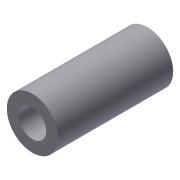
# Autodesk Inventor part: Toughbox Spacers
Saved by Autodesk Inventor 2011 (Build 150239000, 239)
## iProperties
Created: 2012-06-04
Part Number: Toughbox Spacers
Material: Aluminum-6061
Document SubType Name: Modeling
Designer: Nemo
Mass: 7.15711 g
Surface Area: 19.1779 cm^2
Volume: 2.641 cm^3
Density: 2.71 g/cm^3
Author: Nemo
Autodesk Inventor part; units mm, degrees
ref_plane "YZ Plane" through (0, 0, 0) normal (1, 0, 0) x (0, 1, 0)
ref_plane "XZ Plane" through (0, 0, 0) normal (0, 1, 0) x (-1, 0, 0)
ref_plane "XY Plane" through (0, 0, 0) normal (0, 0, 1) x (1, 0, 0)
sketch "Sketch1" plane through (0, 0, 0) normal (0, 0, 1) x (1, 0, 0)
  circle A0 centre (0, 0) radius 3.429
  circle A1 centre (0, 0) radius 6.35
  dimension "d0" = 6.858
  dimension "d1" = 12.7
  constraints: 2 centre point, 2 coincident
  measures "d0" diameter of A0
  measures "d1" diameter of A1
extrude "Extrusion1" add sketch "Sketch1" along normal blind 28.575
body "Solid1"
